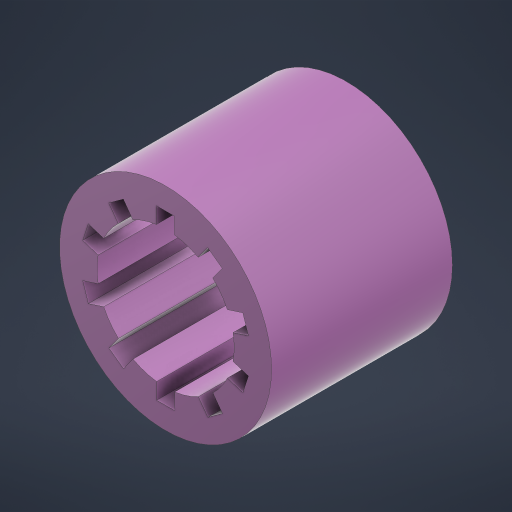
# Autodesk Inventor part: opona
Saved by Autodesk Inventor 2024 (Build 280153000, 153)
## iProperties
Created: 2024-05-24
Part Number: opona
Material: Generic
Document SubType Name: Modeling
Designer: Adam
Density: 1 g/cm^3
Appearance: Default
Author: Adam
Autodesk Inventor part; units mm, degrees
ref_plane "YZ Plane" through (0, 0, 0) normal (1, 0, 0) x (0, 1, 0)
ref_plane "XZ Plane" through (0, 0, 0) normal (0, 1, 0) x (-1, 0, 0)
ref_plane "XY Plane" through (0, 0, 0) normal (0, 0, 1) x (1, 0, 0)
sketch "Sketch1" plane through (0, 0, 0) normal (0, 0, 1) x (1, 0, 0)
  arc A0 (-10.8205, 1.9793) -> (-10.8147, -2.0103) centre (0, 0) ccw
  line L0 (-10.8147, -2.0103) -> (-13.2812, -2.8117)
  line L1 (-12.3877, -5.5615) -> (-13.2812, -2.8117)
  line L2 (-13.2812, -2.8117) -> (-12.3877, -5.5615)
  line L3 (-12.3877, -5.5615) -> (-9.9173, -4.7588)
  line L4 (-12.3974, 5.5317) -> (-13.2908, 2.782)
  line L5 (-13.2908, 2.782) -> (-10.8205, 1.9793)
  line L6 (-9.931, 4.7303) -> (-12.3974, 5.5317)
  arc A1 (-7.5905, 7.9614) -> (-9.931, 4.7303) centre (0, 0) ccw
  line L7 (-6.7782, 11.7623) -> (-9.1173, 10.0628)
  line L8 (-9.1173, 10.0628) -> (-7.5905, 7.9614)
  line L9 (-5.2539, 9.6642) -> (-6.7782, 11.7623)
  arc A2 (-1.4613, 10.9025) -> (-5.2539, 9.6642) centre (0, 0) ccw
  line L10 (1.43, 13.5) -> (-1.4613, 13.5)
  line L11 (-1.4613, 13.5) -> (-1.4613, 10.9025)
  line L12 (1.43, 10.9067) -> (1.43, 13.5)
  arc A3 (5.2261, 9.6792) -> (1.43, 10.9067) centre (0, 0) ccw
  line L13 (9.092, 10.0812) -> (6.7529, 11.7806)
  line L14 (6.7529, 11.7806) -> (5.2261, 9.6792)
  line L15 (7.5677, 7.9831) -> (9.092, 10.0812)
  arc A4 (9.9173, 4.7588) -> (7.5677, 7.9831) centre (0, 0) ccw
  line L16 (13.2812, 2.8117) -> (12.3877, 5.5615)
  line L17 (12.3877, 5.5615) -> (9.9173, 4.7588)
  line L18 (10.8147, 2.0103) -> (13.2812, 2.8117)
  arc A5 (10.8205, -1.9793) -> (10.8147, 2.0103) centre (0, 0) ccw
  line L19 (12.3974, -5.5317) -> (13.2908, -2.782)
  line L20 (13.2908, -2.782) -> (10.8205, -1.9793)
  line L21 (9.931, -4.7303) -> (12.3974, -5.5317)
  arc A6 (7.5905, -7.9614) -> (9.931, -4.7303) centre (0, 0) ccw
  line L22 (6.7782, -11.7623) -> (9.1173, -10.0628)
  line L23 (9.1173, -10.0628) -> (7.5905, -7.9614)
  line L24 (5.2539, -9.6642) -> (6.7782, -11.7623)
  arc A7 (1.4613, -10.9025) -> (5.2539, -9.6642) centre (0, 0) ccw
  line L25 (-1.43, -13.5) -> (1.4613, -13.5)
  line L26 (1.4613, -13.5) -> (1.4613, -10.9025)
  line L27 (-1.43, -10.9067) -> (-1.43, -13.5)
  arc A8 (-5.2261, -9.6792) -> (-1.43, -10.9067) centre (0, 0) ccw
  line L28 (-9.092, -10.0812) -> (-6.7529, -11.7806)
  line L29 (-6.7529, -11.7806) -> (-5.2261, -9.6792)
  line L30 (-7.5677, -7.9831) -> (-9.092, -10.0812)
  arc A9 (-9.9173, -4.7588) -> (-7.5677, -7.9831) centre (0, 0) ccw
  circle A10 centre (0, 0) radius 17
  circle A11 centre (0, 0) radius 8.5
  point P0 (-10.8205, 1.9793)
  point P1 (-7.5905, 7.9614)
  point P2 (5.2261, 9.6792)
  point P3 (9.9173, 4.7588)
  point P4 (10.8205, -1.9793)
  point P5 (7.5905, -7.9614)
  point P6 (1.4613, -10.9025)
  point P7 (-5.2261, -9.6792)
  point P8 (-9.9173, -4.7588)
  dimension "d2" = 360
  dimension "d3" = 34
  dimension "d6" = 11
  dimension "d7" = 17
  dimension "d8" = 2.5933
  dimension "d9" = 2.8912
  constraints: 62 end point, 20 point on circle, 12 centre point, 5 coincident, 2 perpendicular, 101 other
  measures "d3" diameter of A10
  measures "d6" radius of A1
  measures "d7" diameter of A11
  measures "d8" distance of L12.start L10.start
  measures "d9" distance of L10.start L11.start
extrude "Extrusion1" add sketch "Sketch1" along normal blind 29 contours A10
body "Solid1"
